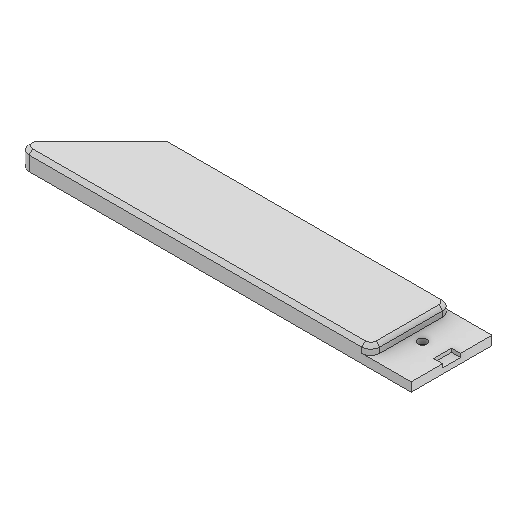
# Autodesk Inventor part: Border
Saved by Autodesk Inventor 2025.2 (Build 292293000, 293)
## iProperties
Created: 2025-03-03
Part Number: Border
Material: Generic
Document SubType Name: Modeling
Designer: Marcu
Density: 1 g/cm^3
Appearance: Default
Author: Marcu
Autodesk Inventor part; units mm, degrees
ref_plane "YZ Plane" through (0, 0, 0) normal (1, 0, 0) x (0, 1, 0)
ref_plane "XZ Plane" through (0, 0, 0) normal (0, 1, 0) x (-1, 0, 0)
ref_plane "XY Plane" through (0, 0, 0) normal (0, 0, 1) x (1, 0, 0)
sketch "Sketch1" plane through (0, 0, 0) normal (0, 0, 1) x (1, 0, 0)
  line L0 (-180, 0) -> (0, 0)
  line L1 (-225, -45) -> (0, -45)
  line L2 (-180, 0) -> (-225, -45)
  line L3 (0, 0) -> (0, -45)
  dimension "d2" = 45
  dimension "d9" = 225
  dimension "d10" = 180
  constraints: 8 end point, 1 horizontal, 1 parallel
  measures "d2" distance between parallel lines of L0 L1
  measures "d9" distance of L1.start L1.end
  measures "d10" distance of L0.start point (0, 0)
extrude "Extrusion1" add sketch "Sketch1" along normal blind 10
sketch "Sketch2" plane through (0, 0, 10) normal (0, 0, 1) x (1, 0, 0)
  line L0 (0, 0) -> (-180, 0) projected
  line L1 (-225, -45) -> (0, -45) projected
  line L2 (0, 0) -> (-22.5, 0)
  line L3 (-22.5, 0) -> (-22.5, -45)
  line L4 (-22.5, -45) -> (0, -45)
  line L5 (0, -45) -> (0, 0)
  dimension "d11" = 22.5
  constraints: 8 end point, 2 parallel, 1 horizontal, 1 perpendicular, 1 point on line
  measures "d11" distance of L4.end L3.end
extrude "Extrusion2" cut sketch "Sketch2" against normal blind 5
sketch "Sketch3" plane through (0, 0, 5) normal (0, 0, 1) x (1, 0, 0)
  line L0 (-5, -17.5) -> (0, -17.5)
  line L1 (0, -27.5) -> (-5, -27.5)
  line L2 (-5, -17.5) -> (-5, -27.5)
  line L3 (0, -17.5) -> (0, -27.5)
  line L4 (0, -45) -> (-22.5, -45) projected
  point P0 (-2.5, -27.5)
  point P1 (0, -22.5)
  dimension "d14" = 5
  dimension "d17" = 10
  dimension "d18" = 22.5
  constraints: 8 end point, 2 midpoint, 1 perpendicular, 1 vertical
  measures "d14" distance of L0.start L0.end
  measures "d17" distance from line of point (-2.5, -27.5) L0
  measures "d18" distance from line of L4 point (0, -22.5)
extrude "Extrusion3" cut sketch "Sketch3" against normal blind 2
sketch "Sketch4" plane through (0, 0, 0) normal (0, 0, -1) x (-1, 0, 0)
  circle A0 centre (22.5, -22.5) radius 7.5
  circle A1 centre (157.5, -22.5) radius 7.5
  point P0 (0, -45)
  point P1 (180, 0)
  dimension "d26" = 15
  dimension "d30" = 15
  constraints: 2 centre point
  measures "d26" diameter of A0
  measures "d30" diameter of A1
extrude "Extrusion4" add sketch "Sketch4" along normal blind 10
fillet "Fillet4" radius 5 4 edges at (-225, -45, 5) (-180, 0, 5) (-22.5, 0, 7.5) (-22.5, -45, 7.5)
chamfer "Chamfer2" distance 2 angle 45 8 edges at (-120.2145, -45, 10) (-23.9645, -43.5355, 10) (-22.5, -22.5, 10) (-23.9645, -1.4645, 10) (-102.7145, 0, 10) (-179.8423, -0.3806, 10) (-198.9645, -18.9645, 10) (-217.5483, -41.9134, 10)
sketch "Sketch5" plane through (0, 0, 5) normal (0, 0, 1) x (1, 0, 0)
  line L0 (-22.5, -40) -> (-22.5, -5) projected
  circle A0 centre (-16.25, -22.5) radius 2.5
  line L1 (0, -45) -> (-27.5, -45) projected
  point P0 (0, 0)
  dimension "d38" = 5
  dimension "d39" = 6.25
  dimension "d40" = 22.5
  constraints: 1 centre point
  measures "d38" diameter of A0
  measures "d39" distance from line of L0 A0.centre
  measures "d40" distance from line of L1 A0.centre
extrude "Extrusion5" cut sketch "Sketch5" against normal blind 3
body "Solid1"
